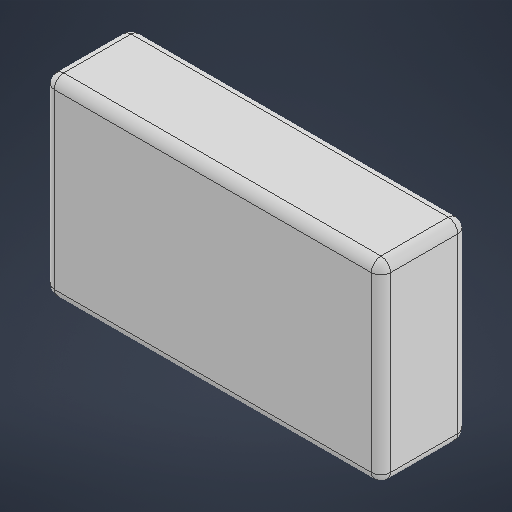
# Autodesk Inventor part: bateria
Saved by Autodesk Inventor 2026.2 (Build 302298010, 298A)
## iProperties
Created: 2026-04-26
Part Number: bateria
Material: Genérico
Document SubType Name: Modeling
Designer: Lucas David
Density: 1 g/cm^3
Appearance: Padrão
Author: Lucas David
Autodesk Inventor part; units mm, degrees
ref_plane "YZ Plane" through (0, 0, 0) normal (1, 0, 0) x (0, 1, 0)
ref_plane "XZ Plane" through (0, 0, 0) normal (0, 1, 0) x (-1, 0, 0)
ref_plane "XY Plane" through (0, 0, 0) normal (0, 0, 1) x (1, 0, 0)
sketch "Esboço1" plane through (0, 0, 0) normal (0, 0, 1) x (1, 0, 0)
  line L0 (-35, -20) -> (35, -20)
  line L1 (35, -20) -> (35, 20)
  line L2 (35, 20) -> (-35, 20)
  line L3 (-35, 20) -> (-35, -20)
  line L4 (-35, -20) -> (35, 20) construction
  line L5 (35, -20) -> (-35, 20) construction
  point P0 (0, 0)
  dimension "d0" = 40
  dimension "d1" = 70
  constraints: 12 end point, 2 midpoint, 2 parallel, 1 horizontal, 1 perpendicular
  measures "d0" distance between parallel lines of L0 L2
  measures "d1" distance between parallel lines of L1 L3
extrude "Extrusão1" add sketch "Esboço1" along normal blind 18
fillet "Arredondamento1" radius 2 12 edges at (0, -20, 18) (0, -20, 0) (0, 20, 0) (0, 20, 18) (35, 20, 9) (35, 0, 18) (35, -20, 9) (35, 0, 0) (-35, -20, 9) (-35, 0, 18) (-35, 0, 0) (-35, 20, 9)
